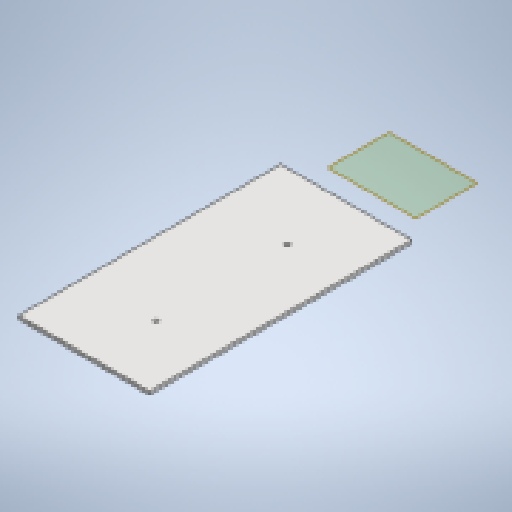
# Autodesk Inventor part: Plate
Saved by Autodesk Inventor 2023.1 (Build 271208000, 208)
## iProperties
Created: 2022-12-24
Part Number: Plate
Material: Generic
Document SubType Name: Modeling
Designer: USER
Density: 1 g/cm^3
Appearance: Default
Author: USER
Autodesk Inventor part; units mm, degrees
ref_plane "YZ Plane" through (0, 0, 0) normal (1, 0, 0) x (0, 1, 0)
ref_plane "XZ Plane" through (0, 0, 0) normal (0, 1, 0) x (-1, 0, 0)
ref_plane "XY Plane" through (0, 0, 0) normal (0, 0, 1) x (1, 0, 0)
ref_plane "Work Plane1" through (70.0345, 2.6931, 201.8136) normal (0, -1, 0) x (1, 0, 0)
sketch "Sketch1" plane through (70.0345, 2.6931, 201.8136) normal (0, -1, 0) x (1, 0, 0)
  line L0 (-70.2433, 298.8217) -> (54.7567, 298.8217)
  line L1 (54.7567, 298.8217) -> (54.7567, 48.8217)
  line L2 (54.7567, 48.8217) -> (-70.2433, 48.8217)
  line L3 (-70.2433, 48.8217) -> (-70.2433, 298.8217)
  circle A0 centre (-0.3511, 237.4444) radius 2.5
  circle A1 centre (-0.6937, 111.9449) radius 2.5
  point P0 (-70.0345, -201.8136)
  dimension "d0" = 125
  dimension "d1" = 250
  dimension "d2" = 5
  dimension "d3" = 5
  dimension "d4" = 125.5
  constraints: 8 end point, 2 centre point, 2 parallel, 1 horizontal, 1 perpendicular
  measures "d0" distance of L1.end L2.end
  measures "d1" distance of L0.end L1.end
  measures "d2" diameter of A0
  measures "d3" diameter of A1
  measures "d4" distance of A1.centre A0.centre
extrude "Extrusion1" add sketch "Sketch1" along normal blind 3
body "Solid1"
